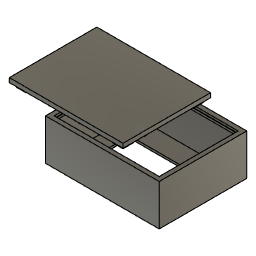
oled v17 (Autodesk Fusion 360 design; units mm, degrees)
Autodesk Fusion 360 part; units mm, degrees
sketch "Sketch1" plane through (0, 0, 0) normal (0, 0, 1) x (1, 0, 0)
  line L0 (0, 0) -> (34.6, 0)
  line L1 (34.6, 0) -> (34.6, 18.5)
  line L2 (34.6, 18.5) -> (0, 18.5)
  line L3 (0, 18.5) -> (0, 0)
  line L4 (0, 18.5) -> (0, 24) construction
  line L5 (0, 0) -> (0, -9.5) construction
  line L6 (0, 14) -> (-2, 14) construction
  line L7 (34.6, 13.1015) -> (36.6, 13.1015) construction
  line L8 (0, 24) -> (39, 24)
  line L9 (36.6, 13.1015) -> (36.6, 24)
  line L10 (0, -9.5) -> (45, -9.5)
  line L11 (0, -9.5) -> (-1, -9.5)
  line L12 (-1, -9.5) -> (-8, -9.5)
  line L13 (36.6, 13.1015) -> (36.6, -9.5)
  line L14 (-2, 14) -> (-2, 25.7073)
  line L15 (-2, 14) -> (-2, -11)
  line L16 (-2, 24) -> (0, 24)
  dimension "d3" = 34.6
  dimension "d4" = 18.5
  dimension "d5" = 5.5
  dimension "d6" = 9.5
  dimension "d7" = 2
  constraint horizontal L0
  constraint vertical L1
  constraint horizontal L2
  constraint vertical L3
  constraint coincident L0.start L3.end
  constraint perpendicular L2 L4
  constraint perpendicular L0 L5
  constraint coincident L3 L6.start
  constraint perpendicular L3 L6
  constraint coincident L1 L7.start
  constraint perpendicular L1 L7
  constraint perpendicular L4 L8
  constraint coincident L8 L9.end
  constraint perpendicular L8 L9
  constraint perpendicular L5 L10
  constraint perpendicular L5 L11
  constraint perpendicular L5 L12
  constraint coincident L10 L13.end
  constraint perpendicular L10 L13
  constraint perpendicular L6 L14
  constraint perpendicular L12 L15
  constraint coincident L14 L16.start
  constraint perpendicular L4 L16
  measures "d3" distance of L0.start L0.end
  measures "d4" distance of L0.start L2.end
  measures "d5" distance of L2.end L4.end
  measures "d6" distance of L0.start L5.end
  measures "d7" distance of L7.start L7.end
extrude "Extrude1" add sketch "Sketch1" along normal blind 1 makes body 1
sketch "Sketch2" plane through (0, 0, 1) normal (0, 0, 1) x (-1, 0, 0)
  line L0 (0, 0) -> (0, -18.5)
  line L1 (0, -18.5) -> (-34.6, -18.5)
  line L2 (-34.6, -18.5) -> (-34.6, 0)
  line L3 (-34.6, 0) -> (0, 0)
  line L4 (2, -24) -> (2, 9.5)
  line L5 (2, 9.5) -> (-36.6, 9.5)
  line L6 (-36.6, 9.5) -> (-36.6, -24)
  line L7 (-36.6, -24) -> (2, -24)
  circle A0 centre (-1.9, -21.7) radius 2.25
  circle A1 centre (-32.3, -21.7) radius 2.25
  line L8 (-1.9, -21.7) -> (-32.3, -21.7) construction
  circle A2 centre (-1.9, 6.8694) radius 2.25
  circle A3 centre (-32.3, 6.8694) radius 2.25
  line L9 (-1.9, 6.8694) -> (-32.3, 6.8694)
  line L10 (-1.9, -21.7) -> (-1.9, 18) construction
  dimension "d10" = 4.5
  dimension "d11" = 4.5
  dimension "d12" = 30.4
  dimension "d13" = 4.5
  dimension "d14" = 4.5
  dimension "d15" = 30.4
  constraint coincident A0.centre L8.start
  constraint horizontal L8
  constraint coincident A1.centre L8.end
  constraint coincident A2.centre L9.start
  constraint horizontal L9
  constraint coincident A3.centre L9.end
  constraint perpendicular L8 L10
  constraint coincident A2.centre L10
  measures "d10" diameter of A0
  measures "d11" diameter of A1
  measures "d12" distance of A0.centre A1.centre
  measures "d13" diameter of A2
  measures "d14" diameter of A3
  measures "d15" distance of A2.centre A3.centre
extrude "Extrude2" add sketch "Sketch2" along normal blind 1.2 contours A0 | A1 | A2 | A3 bodies 1
sketch "Sketch3" plane through (0, 0, 2.2) normal (0, 0, 1) x (-1, 0, 0)
  circle A0 centre (-1.9, -21.7) radius 2.25
  circle A1 centre (-1.9, -21.7) radius 1.55
  dimension "d18" = 3.1
  constraint concentric A0 A1
  measures "d18" diameter of A1
extrude "Extrude3" add sketch "Sketch3" along normal blind 2 contours A1 bodies 1
sketch "Sketch4" plane through (0, 0, 2.2) normal (0, 0, 1) x (-1, 0, 0)
  circle A0 centre (-32.3, -21.7) radius 2.25
  circle A1 centre (-32.3, -21.7) radius 1.55
  dimension "d21" = 3.1
  constraint concentric A0 A1
  measures "d21" diameter of A1
extrude "Extrude4" add sketch "Sketch4" along normal blind 2 contours A1 bodies 1
sketch "Sketch5" plane through (0, 0, 2.2) normal (0, 0, 1) x (-1, 0, 0)
  circle A0 centre (-1.9, 6.8694) radius 2.25
  circle A1 centre (-1.9, 6.8694) radius 1.55
  dimension "d24" = 3.1
  constraint concentric A0 A1
  measures "d24" diameter of A1
extrude "Extrude5" add sketch "Sketch5" along normal blind 2 contours A1 bodies 1
sketch "Sketch6" plane through (0, 0, 2.2) normal (0, 0, 1) x (-1, 0, 0)
  circle A0 centre (-32.3, 6.8694) radius 2.25
  circle A1 centre (-32.3, 6.8694) radius 1.55
  dimension "d27" = 3.1
  constraint concentric A0 A1
  measures "d27" diameter of A1
extrude "Extrude6" add sketch "Sketch6" along normal blind 2 contours A1 bodies 1
sketch "Sketch7" plane through (0, 0, 0) normal (1, 0, 0) x (0, 1, 0)
  line L0 (0, 0) -> (18.5, 0)
  line L1 (18.5, 0) -> (18.5, 1)
  line L2 (18.5, 1) -> (0, 1)
  line L3 (0, 1) -> (0, 0)
extrude "Extrude7" add sketch "Sketch7" along normal blind 0.5 bodies 1
sketch "Sketch8" plane through (34.6, 0, 0) normal (-1, 0, 0) x (0, -1, 0)
  line L0 (-18.5, 0) -> (0, 0)
  line L1 (0, 0) -> (0, 1)
  line L2 (0, 1) -> (-18.5, 1)
  line L3 (-18.5, 1) -> (-18.5, 0)
extrude "Extrude8" add sketch "Sketch8" along normal blind 0.5 bodies 1
sketch "Sketch9" plane through (0, 18.5, 0) normal (0, -1, 0) x (1, 0, 0)
  line L0 (34.1, 0) -> (34.1, 1)
  line L1 (34.1, 1) -> (0.5, 1)
  line L2 (0.5, 1) -> (0.5, 0)
  line L3 (0.5, 0) -> (34.1, 0)
extrude "Extrude9" add sketch "Sketch9" along normal blind 0.5 bodies 1
sketch "Sketch10" plane through (0, 0, 4.2) normal (0, 0, 1) x (-1, 0, 0)
  circle A0 centre (-32.3, -21.7) radius 1.55
extrude "Extrude10" cut sketch "Sketch10" against normal blind 2 bodies 1
sketch "Sketch11" plane through (0, 0, 4.2) normal (0, 0, 1) x (-1, 0, 0)
  circle A0 centre (-1.9, -21.7) radius 1.55
extrude "Extrude11" cut sketch "Sketch11" against normal blind 2 bodies 1
sketch "Sketch12" plane through (0, 0, 4.2) normal (0, 0, 1) x (-1, 0, 0)
  circle A0 centre (-1.9, 6.8694) radius 1.55
extrude "Extrude12" cut sketch "Sketch12" against normal blind 2 bodies 1
sketch "Sketch13" plane through (0, 0, 4.2) normal (0, 0, 1) x (-1, 0, 0)
  circle A0 centre (-32.3, 6.8694) radius 1.55
extrude "Extrude13" cut sketch "Sketch13" against normal blind 2 bodies 1
sketch "Sketch14" plane through (0, 0, 2.2) normal (0, 0, 1) x (-1, 0, 0)
  circle A0 centre (-1.9, -21.7) radius 2.25
sketch "Sketch15" plane through (0, 0, 2.2) normal (0, 0, 1) x (-1, 0, 0)
  circle A0 centre (-32.3, -21.7) radius 2.25
  circle A1 centre (-32.3, -21.7) radius 1.625
  dimension "d44" = 3.25
  constraint concentric A0 A1
  measures "d44" diameter of A1
extrude "Extrude14" add sketch "Sketch15" along normal blind 2 contours A1 bodies 1
sketch "Sketch16" plane through (0, 0, 2.2) normal (0, 0, 1) x (-1, 0, 0)
  circle A0 centre (-32.3, 6.8694) radius 2.25
  circle A1 centre (-32.3, 6.8694) radius 1.625
  dimension "d47" = 3.25
  constraint concentric A0 A1
  measures "d47" diameter of A1
extrude "Extrude15" add sketch "Sketch16" along normal blind 2 contours A1 bodies 1
sketch "Sketch17" plane through (0, 0, 2.2) normal (0, 0, 1) x (-1, 0, 0)
  circle A0 centre (-1.9, 6.8694) radius 2.25
  circle A1 centre (-1.9, 6.8694) radius 1.625
  dimension "d50" = 3.25
  constraint concentric A0 A1
  measures "d50" diameter of A1
extrude "Extrude16" add sketch "Sketch17" along normal blind 2 contours A1 bodies 1
sketch "Sketch18" plane through (0, 0, 2.2) normal (0, 0, 1) x (1, 0, 0)
  circle A0 centre (1.883, 21.7106) radius 1.625
  dimension "d53" = 3.25
  measures "d53" diameter of A0
extrude "Extrude17" add sketch "Sketch18" along normal blind 2 bodies 1
sketch "Sketch19" plane through (-2, 0, 0) normal (-1, 0, 0) x (0, -1, 0)
  line L0 (-24, 0) -> (9.5, 0)
  line L1 (9.5, 0) -> (9.5, 1)
  line L2 (9.5, 1) -> (-24, 1)
  line L3 (-24, 1) -> (-24, 0)
extrude "Extrude18" add sketch "Sketch19" along normal blind 9 bodies 1
sketch "Sketch20" plane through (36.6, 0, 0) normal (1, 0, 0) x (0, 1, 0)
  line L0 (-9.5, 0) -> (24, 0)
  line L1 (24, 0) -> (24, 1)
  line L2 (24, 1) -> (-9.5, 1)
  line L3 (-9.5, 1) -> (-9.5, 0)
extrude "Extrude19" add sketch "Sketch20" along normal blind 9 bodies 1
sketch "Sketch21" plane through (0, 24, 0) normal (0, 1, 0) x (-1, 0, 0)
  line L0 (-45.6, 0) -> (11, 0)
  line L1 (11, 0) -> (11, 1)
  line L2 (11, 1) -> (-45.6, 1)
  line L3 (-45.6, 1) -> (-45.6, 0)
extrude "Extrude20" add sketch "Sketch21" along normal blind 3 bodies 1
move_face "OffsetFaces1" offset -2 1 faces at (-11, 14.8333, 0.6667) on bodies 1
move_face "OffsetFaces2" offset -2 1 faces at (45.6, 2.6667, 0.6667) on bodies 1
sketch "Sketch22" plane through (0, 0, 0) normal (0, 0, -1) x (1, 0, 0)
  line L0 (0.5, -18) -> (0.5, 0)
  line L1 (0.5, 0) -> (34.1, 0)
  line L2 (34.1, 0) -> (34.1, -18)
  line L3 (34.1, -18) -> (0.5, -18)
  line L4 (43.6, -27) -> (43.6, 9.5)
  line L5 (43.6, 9.5) -> (-9, 9.5)
  line L6 (-9, 9.5) -> (-9, -27)
  line L7 (-9, -27) -> (43.6, -27)
  line L8 (45.6, -29) -> (45.6, 11.5)
  line L9 (45.6, 11.5) -> (-11, 11.5)
  line L10 (-11, 11.5) -> (-11, -29)
  line L11 (-11, -29) -> (45.6, -29)
  dimension "d64" = 2
extrude "Extrude21" add sketch "Sketch22" against normal blind 16 contours L8 L9 L10 L11 bodies 1
sketch "Sketch23" plane through (-11, 0, 0) normal (-1, 0, 0) x (0, -1, 0)
  line L0 (-29, 0) -> (11.5, 0)
  line L1 (11.5, 0) -> (11.5, 16)
  line L2 (11.5, 16) -> (-29, 16)
  line L3 (-29, 16) -> (-29, 0)
  line L4 (-16, 8) -> (-7, 8)
  line L5 (-16, 8) -> (-16, 16)
  line L6 (-7, 8) -> (-7, 16)
  constraint coincident L2 L5.end
  constraint perpendicular L2 L5
  constraint coincident L2 L6.end
  constraint perpendicular L2 L6
extrude "Extrude22" cut sketch "Sketch23" against normal blind 2 contours L2 L4 L5 L6 bodies 1
move_face "OffsetFaces3" offset 2 1 faces at (-9, -4, 8.3333) on bodies 1
sketch "Sketch24" plane through (-11, 0, 0) normal (-1, 0, 0) x (0, -1, 0)
  line L0 (-16, 8) -> (-16, 16)
  line L1 (-16, 16) -> (-29, 16)
  line L2 (-29, 16) -> (-29, 0)
  line L3 (-29, 0) -> (11.5, 0)
  line L4 (11.5, 0) -> (11.5, 16)
  line L5 (11.5, 16) -> (-7, 16)
  line L6 (-7, 16) -> (-7, 8)
  line L7 (-7, 8) -> (-16, 8)
extrude "Extrude23" cut sketch "Sketch24" against normal blind 1.99 bodies 1
move_face "OffsetFaces4" offset 2 1 faces at (43.6, 14.8333, 11) on bodies 1
sketch "Sketch25" plane through (45.6, 0, 0) normal (1, 0, 0) x (0, 1, 0)
  line L0 (-11.5, 0) -> (29, 0)
  line L1 (29, 0) -> (29, 16)
  line L2 (29, 16) -> (-11.5, 16)
  line L3 (-11.5, 16) -> (-11.5, 0)
extrude "Extrude24" cut sketch "Sketch25" against normal blind 2 bodies 1
sketch "Sketch26" plane through (-7, 0, 0) normal (1, 0, 0) x (0, 1, 0)
  line L0 (16, 16) -> (16, 8)
  line L1 (16, 8) -> (7, 8)
  line L2 (7, 8) -> (7, 16)
  line L3 (7, 16) -> (-9.5, 16)
  line L4 (-9.5, 16) -> (-9.5, 1)
  line L5 (-9.5, 1) -> (27, 1)
  line L6 (27, 1) -> (27, 16)
  line L7 (27, 16) -> (16, 16)
  line L8 (7, 8) -> (7, 11)
  line L9 (7, 11) -> (2, 11)
  line L10 (16, 8) -> (16, 11)
  line L11 (16, 11) -> (21, 11)
  line L12 (21, 11) -> (21, 13)
  line L13 (21, 13) -> (2, 13)
  line L14 (2, 13) -> (2, 11)
  dimension "d80" = 3
  dimension "d81" = 5
  dimension "d82" = 2
  constraint coincident L1.end L2.start
  constraint perpendicular L1 L8
  constraint perpendicular L8 L9
  constraint coincident L0.end L1.start
  constraint coincident L0 L10.end
  constraint perpendicular L1 L10
  constraint perpendicular L10 L11
  constraint perpendicular L11 L12
  constraint perpendicular L12 L13
  constraint perpendicular L9 L14
  measures "d80" distance of L1.end L8.end
  measures "d81" distance of L10.end L11.end
  measures "d82" distance of L11.end L12.end
extrude "Extrude25" cut sketch "Sketch26" against normal blind 1.6 contours L0 L11 L12 L13 | L2 L9 L13 L14 bodies 1
sketch "Sketch27" plane through (-7, 0, 0) normal (1, 0, 0) x (0, 1, 0)
  line L0 (2, 13) -> (7, 13)
  line L1 (7, 13) -> (7, 16)
  line L2 (7, 16) -> (-9.5, 16)
  line L3 (-9.5, 16) -> (-9.5, 1)
  line L4 (-9.5, 1) -> (27, 1)
  line L5 (27, 1) -> (27, 16)
  line L6 (27, 16) -> (16, 16)
  line L7 (16, 16) -> (16, 13)
  line L8 (16, 13) -> (21, 13)
  line L9 (21, 13) -> (21, 11)
  line L10 (21, 11) -> (16, 11)
  line L11 (16, 11) -> (16, 8)
  line L12 (16, 8) -> (7, 8)
  line L13 (7, 8) -> (7, 11)
  line L14 (7, 11) -> (2, 11)
  line L15 (2, 11) -> (2, 13)
  line L16 (2, 13) -> (2, 16)
  line L17 (21, 13) -> (21, 16)
  constraint coincident L0.start L15.end
  constraint perpendicular L0 L16
  constraint coincident L8.end L9.start
  constraint coincident L6 L17.end
  constraint perpendicular L6 L17
extrude "Extrude26" cut sketch "Sketch27" against normal blind 2.01 contours L0 L1 L2 L16 | L6 L7 L8 L17 bodies 1
sketch "Sketch28" plane through (-7, 0, 0) normal (1, 0, 0) x (0, 1, 0)
  line L0 (21, 16) -> (21, 11)
  line L1 (21, 11) -> (16, 11)
  line L2 (16, 11) -> (16, 8)
  line L3 (16, 8) -> (7, 8)
  line L4 (7, 8) -> (7, 11)
  line L5 (7, 11) -> (2, 11)
  line L6 (2, 11) -> (2, 16)
  line L7 (2, 16) -> (-9.5, 16)
  line L8 (-9.5, 16) -> (-9.5, 1)
  line L9 (-9.5, 1) -> (27, 1)
  line L10 (27, 1) -> (27, 16)
  line L11 (27, 16) -> (21, 16)
  line L12 (2, 11) -> (2, 10)
  line L13 (2, 10) -> (21, 10)
  line L14 (21, 10) -> (21, 11)
  constraint coincident L5.end L6.start
  constraint perpendicular L5 L12
  constraint perpendicular L12 L13
  constraint coincident L0.end L1.start
extrude "Extrude27" cut sketch "Sketch28" against normal blind 1.6 contours L1 L2 L13 L14 | L4 L5 L12 L13 bodies 1
sketch "Sketch29" plane through (0, 0, 16) normal (0, 0, 1) x (-1, 0, 0)
  line L0 (9.01, -21) -> (7, -21)
  line L1 (7, -21) -> (7, -27)
  line L2 (7, -27) -> (-41.6, -27)
  line L3 (-41.6, -27) -> (-41.6, 9.5)
  line L4 (-41.6, 9.5) -> (7, 9.5)
  line L5 (7, 9.5) -> (7, -2)
  line L6 (7, -2) -> (9.01, -2)
  line L7 (9.01, -2) -> (9.01, 11.5)
  line L8 (9.01, 11.5) -> (-43.6, 11.5)
  line L9 (-43.6, 11.5) -> (-43.6, -29)
  line L10 (-43.6, -29) -> (9.01, -29)
  line L11 (9.01, -29) -> (9.01, -21)
extrude "Extrude28" add sketch "Sketch29" along normal blind 3 bodies 1
copy_body "Body->Comp1" bodies 1 removing the originals makes body 2 in component "Component"
sketch "Sketch1 (2)" plane through (0, 0, 19) normal (0, 0, 1) x (-1, 0, 0) in component "Component'"
  line L0 (9.01, -29) -> (9.01, -21)
  line L1 (9.01, -21) -> (7, -21)
  line L2 (7, -21) -> (7, -27)
  line L3 (7, -27) -> (-41.6, -27)
  line L4 (-41.6, -27) -> (-41.6, 9.5)
  line L5 (-41.6, 9.5) -> (7, 9.5)
  line L6 (7, 9.5) -> (7, -2)
  line L7 (7, -2) -> (9.01, -2)
  line L8 (9.01, -2) -> (9.01, 11.5)
  line L9 (9.01, 11.5) -> (-43.6, 11.5)
  line L10 (-43.6, 11.5) -> (-43.6, -29)
  line L11 (-43.6, -29) -> (9.01, -29)
  line L12 (9.01, -29) -> (-43.6, -29)
  line L13 (-43.6, -29) -> (-43.6, 11.5)
  line L14 (-43.6, 11.5) -> (9.01, 11.5)
  line L15 (9.01, 11.5) -> (9.01, -29)
  constraint horizontal L12
  constraint vertical L13
  constraint horizontal L14
  constraint vertical L15
  constraint coincident L9.end L10.start
  constraint coincident L0.start L11.end
extrude "Extrude1'" add sketch "Sketch1 (2)" along normal blind 2 separate body makes body 3 in component "Component'"
sketch "Sketch2 (2)" plane through (0, 0, 8) normal (0, 0, 1) x (-1, 0, 0) in component "Component'"
  line L0 (9.01, -16) -> (9.01, -7)
  line L1 (9.01, -7) -> (7, -7)
  line L2 (7, -7) -> (7, -16)
  line L3 (7, -16) -> (9.01, -16)
extrude "Extrude2'" add sketch "Sketch2 (2)" along normal blind 6 from surface at 5 bodies 3 in component "Component'"
move_face "OffsetFaces1'" offset 5 1 faces at (-7.67, 16, 15) on bodies 3 in component "Component'"
move_face "OffsetFaces2'" offset 5 1 faces at (-8.34, 7, 15) on bodies 3 in component "Component'"
sketch "Sketch1 (3)" plane through (-7, 0, 0) normal (1, 0, 0) x (0, 1, 0) in component "Component"
  line L0 (2, 10) -> (2, 19)
  line L1 (2, 19) -> (-9.5, 19)
  line L2 (-9.5, 19) -> (-9.5, 1)
  line L3 (-9.5, 1) -> (27, 1)
  line L4 (27, 1) -> (27, 19)
  line L5 (27, 19) -> (21, 19)
  line L6 (21, 19) -> (21, 11)
  line L7 (21, 11) -> (21, 10)
  line L8 (21, 10) -> (16, 10)
  line L9 (16, 10) -> (16, 8)
  line L10 (16, 8) -> (7, 8)
  line L11 (7, 8) -> (7, 10)
  line L12 (7, 10) -> (2, 10)
  line L13 (21, 18) -> (21, 16.8)
  line L14 (21, 18) -> (21.6841, 18)
  line L15 (21.6841, 18) -> (27, 18)
  line L16 (21, 16.8) -> (27, 16.8)
  dimension "d98" = 1.2
  constraint coincident L6 L13.start
  constraint coincident L4 L15.end
  constraint parallel L6 L13
  constraint perpendicular L4 L15
  constraint coincident L4 L16.end
  constraint perpendicular L4 L16
  measures "d98" distance of L13.start L13.end
extrude "Extrude1''" cut sketch "Sketch1 (3)" against normal blind 1 contours L4 L6 L13 L14 L15 L16 bodies 2 in component "Component"
sketch "Sketch2 (3)" plane through (0, 27, 0) normal (0, -1, 0) x (1, 0, 0) in component "Component"
  line L0 (-7, 1) -> (41.6, 1)
  line L1 (41.6, 1) -> (41.6, 19)
  line L2 (41.6, 19) -> (-7, 19)
  line L3 (-7, 19) -> (-7, 18)
  line L4 (-7, 18) -> (-8, 18)
  line L5 (-8, 18) -> (-8, 16.8)
  line L6 (-8, 16.8) -> (-7, 16.8)
  line L7 (-7, 16.8) -> (-7, 1)
  line L8 (-7, 18) -> (42, 18)
  line L9 (-7, 16.8) -> (41.6, 16.8)
  constraint coincident L3.end L4.start
  constraint perpendicular L1 L8
  constraint coincident L6.end L7.start
  constraint coincident L1 L9.end
  constraint perpendicular L1 L9
extrude "Extrude2''" cut sketch "Sketch2 (3)" against normal blind 1 contours L1 L4 L5 L6 L8 L9 bodies 2 in component "Component"
sketch "Sketch3 (2)" plane through (41.6, 0, 0) normal (-1, 0, 0) x (0, -1, 0) in component "Component"
  line L0 (-27, 1) -> (9.5, 1)
  line L1 (9.5, 1) -> (9.5, 19)
  line L2 (9.5, 19) -> (-27, 19)
  line L3 (-27, 19) -> (-27, 18)
  line L4 (-27, 18) -> (-28, 18)
  line L5 (-28, 18) -> (-28, 16.8)
  line L6 (-28, 16.8) -> (-27, 16.8)
  line L7 (-27, 16.8) -> (-27, 1)
  line L8 (-27, 18) -> (9.5, 18)
  line L9 (-27, 16.8) -> (9.5, 16.8)
  constraint coincident L3.end L4.start
  constraint coincident L1 L8.end
  constraint perpendicular L1 L8
  constraint coincident L6.end L7.start
  constraint coincident L1 L9.end
  constraint perpendicular L1 L9
extrude "Extrude3'" cut sketch "Sketch3 (2)" against normal blind 1 contours L1 L4 L5 L6 L8 L9 bodies 2 in component "Component"
sketch "Sketch4 (2)" plane through (0, -9.5, 0) normal (0, 1, 0) x (-1, 0, 0) in component "Component"
  line L0 (-41.6, 1) -> (7, 1)
  line L1 (7, 1) -> (7, 19)
  line L2 (7, 19) -> (-41.6, 19)
  line L3 (-41.6, 19) -> (-41.6, 18)
  line L4 (-41.6, 18) -> (-42.6, 18)
  line L5 (-42.6, 18) -> (-42.6, 16.8)
  line L6 (-42.6, 16.8) -> (-41.6, 16.8)
  line L7 (-41.6, 16.8) -> (-41.6, 1)
  line L8 (-41.6, 16.8) -> (7, 16.8)
  line L9 (-41.6, 18) -> (7, 18)
  constraint coincident L6.end L7.start
  constraint coincident L1 L8.end
  constraint perpendicular L1 L8
  constraint coincident L3.end L4.start
  constraint coincident L1 L9.end
  constraint perpendicular L1 L9
extrude "Extrude4'" cut sketch "Sketch4 (2)" against normal blind 1 contours L1 L4 L5 L6 L8 L9 bodies 2 in component "Component"
sketch "Sketch5 (2)" plane through (-7, 0, 0) normal (1, 0, 0) x (0, 1, 0) in component "Component"
  line L0 (27, 16.8) -> (21, 16.8)
  line L1 (21, 16.8) -> (21, 11)
  line L2 (21, 11) -> (21, 10)
  line L3 (21, 10) -> (16, 10)
  line L4 (16, 10) -> (16, 8)
  line L5 (16, 8) -> (7, 8)
  line L6 (7, 8) -> (7, 10)
  line L7 (7, 10) -> (2, 10)
  line L8 (2, 10) -> (2, 19)
  line L9 (2, 19) -> (-9.5, 19)
  line L10 (-9.5, 19) -> (-9.5, 18)
  line L11 (-9.5, 18) -> (-10.5, 18)
  line L12 (-10.5, 18) -> (-10.5, 16.8)
  line L13 (-10.5, 16.8) -> (-9.5, 16.8)
  line L14 (-9.5, 16.8) -> (-9.5, 1)
  line L15 (-9.5, 1) -> (27, 1)
  line L16 (27, 1) -> (27, 16.8)
  line L17 (-9.5, 16.8) -> (2, 16.8)
  line L18 (-9.5, 18) -> (2, 18)
  constraint coincident L13.end L14.start
  constraint coincident L8 L17.end
  constraint perpendicular L8 L17
  constraint coincident L10.end L11.start
  constraint coincident L8 L18.end
  constraint perpendicular L8 L18
extrude "Extrude5'" cut sketch "Sketch5 (2)" against normal blind 1 contours L8 L11 L12 L13 L17 L18 bodies 2 in component "Component"
sketch "Sketch3 (3)" plane through (0, 0, 19) normal (0, 0, -1) x (1, 0, 0) in component "Component'"
  line L0 (-7, -21) -> (-9.01, -21)
  line L1 (-9.01, -21) -> (-9.01, -29)
  line L2 (-9.01, -29) -> (43.6, -29)
  line L3 (43.6, -29) -> (43.6, 11.5)
  line L4 (43.6, 11.5) -> (-9.01, 11.5)
  line L5 (-9.01, 11.5) -> (-9.01, -2)
  line L6 (-9.01, -2) -> (-7, -2)
  line L7 (-7, -2) -> (-7, -21)
  line L8 (-7, 9.5) -> (-3, 9.5)
  line L9 (-3, 9.5) -> (-3, 5.5)
  line L10 (-3, 5.5) -> (-7, 5.5)
  line L11 (-7, 5.5) -> (-7, 9.5)
  dimension "d109" = 4
  dimension "d110" = 4
  constraint horizontal L8
  constraint vertical L9
  constraint horizontal L10
  constraint vertical L11
  measures "d109" distance of L8.start L8.end
  measures "d110" distance of L8.start L10.end
extrude "Extrude3''" add sketch "Sketch3 (3)" along normal blind 2.2 contours L8 L9 L10 L11 bodies 3 in component "Component'"
sketch "Sketch4 (3)" plane through (-7, 0, 0) normal (-1, 0, 0) x (0, -1, 0) in component "Component'"
  line L0 (9.5, 19) -> (5.5, 19)
  line L1 (5.5, 19) -> (5.5, 16.8)
  line L2 (5.5, 16.8) -> (9.5, 16.8)
  line L3 (9.5, 16.8) -> (9.5, 19)
  line L4 (9.5, 16.8) -> (9.5, 17.7)
  line L5 (5.5, 16.8) -> (5.5, 17.7)
  line L6 (5.5, 17.7) -> (9.5, 17.7)
  constraint coincident L2.end L3.start
  constraint coincident L3 L4.end
  constraint perpendicular L2 L4
  constraint coincident L1.end L2.start
  constraint coincident L1 L5.end
  constraint perpendicular L2 L5
  constraint perpendicular L5 L6
extrude "Extrude4''" add sketch "Sketch4 (3)" along normal blind 0.9 contours L1 L2 L3 L4 L5 L6 bodies 3 in component "Component'"
chamfer "Chamfer1" distance 0.9 angle 45 1 edges at (-7.9, -7.5, 16.8) on bodies 3 in component "Component'"
sketch "Sketch5 (3)" plane through (0, -9.5, 0) normal (0, -1, 0) x (1, 0, 0) in component "Component'"
  line L0 (-7.9, 17.7) -> (-7, 16.8)
  line L1 (-7, 16.8) -> (-3, 16.8)
  line L2 (-3, 16.8) -> (-3, 19)
  line L3 (-3, 19) -> (-7, 19)
  line L4 (-7, 19) -> (-7, 17.7)
  line L5 (-7, 17.7) -> (-7.9, 17.7)
  line L6 (-7, 17.7) -> (-3, 17.7)
  line L7 (-7, 17.7) -> (-7, 16.8)
  constraint coincident L4.end L5.start
  constraint coincident L2 L6.end
  constraint perpendicular L2 L6
  constraint coincident L0.end L1.start
extrude "Extrude5''" add sketch "Sketch5 (3)" along normal blind 0.9 contours L1 L2 L6 L7 bodies 3 in component "Component'"
chamfer "Chamfer2" distance 0.9 angle 45 1 edges at (-5, -10.4, 16.8) on bodies 3 in component "Component'"
sketch "Sketch6 (2)" plane through (0, 0, 19) normal (0, 0, -1) x (1, 0, 0) in component "Component'"
  line L0 (-7, 5.5) -> (-7, 9.5)
  line L1 (-7, 9.5) -> (-3, 9.5)
  line L2 (-3, 9.5) -> (-3, 5.5)
  line L3 (-3, 5.5) -> (-7, 5.5)
  line L4 (-7, -21) -> (-9.01, -21)
  line L5 (-9.01, -21) -> (-9.01, -29)
  line L6 (-9.01, -29) -> (43.6, -29)
  line L7 (43.6, -29) -> (43.6, 11.5)
  line L8 (43.6, 11.5) -> (-9.01, 11.5)
  line L9 (-9.01, 11.5) -> (-9.01, -2)
  line L10 (-9.01, -2) -> (-7, -2)
  line L11 (-7, -2) -> (-7, -21)
  line L12 (41.6, 9.5) -> (37.6, 9.5)
  line L13 (37.6, 9.5) -> (37.6, 5.5)
  line L14 (37.6, 5.5) -> (41.6, 5.5)
  line L15 (41.6, 5.5) -> (41.6, 9.5)
  dimension "d119" = 4
  dimension "d120" = 4
  constraint horizontal L12
  constraint vertical L13
  constraint horizontal L14
  constraint vertical L15
  measures "d119" distance of L12.start L12.end
  measures "d120" distance of L12.start L14.end
extrude "Extrude6'" add sketch "Sketch6 (2)" along normal blind 2.2 contours L12 L13 L14 L15 bodies 3 in component "Component'"
sketch "Sketch7 (2)" plane through (41.6, 0, 0) normal (1, 0, 0) x (0, 1, 0) in component "Component'"
  line L0 (-5.5, 19) -> (-9.5, 19)
  line L1 (-9.5, 19) -> (-9.5, 16.8)
  line L2 (-9.5, 16.8) -> (-5.5, 16.8)
  line L3 (-5.5, 16.8) -> (-5.5, 19)
  line L4 (-5.5, 16.8) -> (-5.5, 17.7)
  line L5 (-5.5, 17.7) -> (-9.5, 17.7)
  dimension "d123" = 0.9
  constraint coincident L2.end L3.start
  constraint perpendicular L0 L4
  constraint coincident L1 L5.end
  constraint perpendicular L1 L5
  measures "d123" distance of L2.end L4.end
extrude "Extrude7'" add sketch "Sketch7 (2)" along normal blind 0.9 contours L1 L2 L3 L4 L5 bodies 3 in component "Component'"
chamfer "Chamfer3" distance 0.9 angle 45 1 edges at (42.5, -7.5, 16.8) on bodies 3 in component "Component'"
sketch "Sketch8 (2)" plane through (0, -9.5, 0) normal (0, -1, 0) x (1, 0, 0) in component "Component'"
  line L0 (41.6, 16.8) -> (42.5, 17.7)
  line L1 (42.5, 17.7) -> (41.6, 17.7)
  line L2 (41.6, 17.7) -> (41.6, 19)
  line L3 (41.6, 19) -> (37.6, 19)
  line L4 (37.6, 19) -> (37.6, 16.8)
  line L5 (37.6, 16.8) -> (41.6, 16.8)
  line L6 (41.6, 16.8) -> (41.6, 17.7)
  line L7 (41.6, 17.7) -> (37.6, 17.7)
  constraint coincident L0.start L5.end
  constraint coincident L1.end L2.start
  constraint coincident L4 L7.end
  constraint perpendicular L4 L7
extrude "Extrude8'" add sketch "Sketch8 (2)" along normal blind 0.9 contours L4 L5 L6 L7 bodies 3 in component "Component'"
chamfer "Chamfer4" distance 0.9 angle 45 1 edges at (39.6, -10.4, 16.8) on bodies 3 in component "Component'"
sketch "Sketch9 (2)" plane through (0, 0, 19) normal (0, 0, -1) x (1, 0, 0) in component "Component'"
  line L0 (41.6, 5.5) -> (37.6, 5.5)
  line L1 (37.6, 5.5) -> (37.6, 9.5)
  line L2 (37.6, 9.5) -> (41.6, 9.5)
  line L3 (41.6, 9.5) -> (41.6, 5.5)
  line L4 (-7, 5.5) -> (-7, 9.5)
  line L5 (-7, 9.5) -> (-3, 9.5)
  line L6 (-3, 9.5) -> (-3, 5.5)
  line L7 (-3, 5.5) -> (-7, 5.5)
  line L8 (-7, -21) -> (-9.01, -21)
  line L9 (-9.01, -21) -> (-9.01, -29)
  line L10 (-9.01, -29) -> (43.6, -29)
  line L11 (43.6, -29) -> (43.6, 11.5)
  line L12 (43.6, 11.5) -> (-9.01, 11.5)
  line L13 (-9.01, 11.5) -> (-9.01, -2)
  line L14 (-9.01, -2) -> (-7, -2)
  line L15 (-7, -2) -> (-7, -21)
  line L16 (41.6, -27) -> (37.6, -27)
  line L17 (37.6, -27) -> (37.6, -23)
  line L18 (37.6, -23) -> (41.6, -23)
  line L19 (41.6, -23) -> (41.6, -27)
  dimension "d130" = 4
  dimension "d131" = 4
  constraint horizontal L16
  constraint vertical L17
  constraint horizontal L18
  constraint vertical L19
  measures "d130" distance of L16.start L16.end
  measures "d131" distance of L16.start L18.end
extrude "Extrude9'" add sketch "Sketch9 (2)" along normal blind 2.2 contours L16 L17 L18 L19 bodies 3 in component "Component'"
sketch "Sketch10 (2)" plane through (0, 27, 0) normal (0, 1, 0) x (-1, 0, 0) in component "Component'"
  line L0 (-37.6, 19) -> (-41.6, 19)
  line L1 (-41.6, 19) -> (-41.6, 16.8)
  line L2 (-41.6, 16.8) -> (-37.6, 16.8)
  line L3 (-37.6, 16.8) -> (-37.6, 19)
  line L4 (-37.6, 16.8) -> (-37.6, 17.7)
  line L5 (-37.6, 17.7) -> (-41.6, 17.7)
  dimension "d134" = 0.9
  constraint coincident L2.end L3.start
  constraint perpendicular L2 L4
  constraint coincident L1 L5.end
  constraint perpendicular L1 L5
  measures "d134" distance of L2.end L4.end
extrude "Extrude10'" add sketch "Sketch10 (2)" along normal blind 0.9 contours L1 L2 L3 L4 L5 bodies 3 in component "Component'"
chamfer "Chamfer5" distance 0.9 angle 45 1 edges at (39.6, 27.9, 16.8) on bodies 3 in component "Component'"
sketch "Sketch11 (2)" plane through (41.6, 0, 0) normal (1, 0, 0) x (0, 1, 0) in component "Component'"
  line L0 (27, 16.8) -> (27.9, 17.7)
  line L1 (27.9, 17.7) -> (27, 17.7)
  line L2 (27, 17.7) -> (27, 19)
  line L3 (27, 19) -> (23, 19)
  line L4 (23, 19) -> (23, 16.8)
  line L5 (23, 16.8) -> (27, 16.8)
  line L6 (27, 16.8) -> (27, 17.7)
  line L7 (27, 17.7) -> (23, 17.7)
  constraint coincident L0.start L5.end
  constraint coincident L1.end L2.start
  constraint coincident L4 L7.end
  constraint perpendicular L4 L7
extrude "Extrude11'" add sketch "Sketch11 (2)" along normal blind 0.9 contours L4 L5 L6 L7 bodies 3 in component "Component'"
chamfer "Chamfer6" distance 0.9 angle 45 1 edges at (42.5, 25, 16.8) on bodies 3 in component "Component'"
component "Component" placed x (1, 0, 0) y (0, 1, 0) z (0, 0, 1) at (0, 0, 0)
component "Component'" placed x (1, 0, 0) y (0, 1, 0) z (0, 0, 1) at (0, 0, 0) in component "Component"
